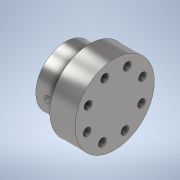
# Autodesk Inventor part: хвостовик
Saved by Autodesk Inventor 2021 (Build 250183000, 183)
## iProperties
Created: 2021-01-19
Part Number: хвостовик
Material: Сталь, легированная
Document SubType Name: ЛистМат
Designer: panda
Density: 7.73 g/cm^3
Sheet Metal Rule: По умолчанию_мм
Appearance: С умеренной полировкой
Mass: 1576.94 g
Surface Area: 253.207 cm^2
Volume: 204.003 cm^3
Author: panda
Autodesk Inventor part; units mm, degrees
ref_plane "YZ Plane" through (0, 0, 0) normal (1, 0, 0) x (0, 1, 0)
ref_plane "XZ Plane" through (0, 0, 0) normal (0, 1, 0) x (-1, 0, 0)
ref_plane "XY Plane" through (0, 0, 0) normal (0, 0, 1) x (1, 0, 0)
sketch "Эскиз1" plane through (0, 0, 0) normal (1, 0, 0) x (0, 1, 0)
  circle A0 centre (0, 0) radius 30.5
  dimension "d0" = 61
  constraints: 1 centre point, 1 coincident
  measures "d0" diameter of A0
extrude "Выдавливание1" add sketch "Эскиз1" along normal blind 25
sketch "Эскиз2" plane through (25, 0, 0) normal (1, 0, 0) x (0, 0, -1)
  circle A0 centre (0, 0) radius 41
  dimension "d3" = 82
  constraints: 1 centre point, 1 coincident
  measures "d3" diameter of A0
extrude "Выдавливание2" add sketch "Эскиз2" along normal blind 26
sketch "Эскиз3" plane through (0, 0, 0) normal (0, 0, 1) x (1, 0, 0)
  line L0 (0, 0) -> (25, 0)
  line L1 (25, -30.5) -> (25, 30.5) projected
  circle A0 centre (12.5, 0) radius 3.5
  dimension "d6" = 7
  constraints: 2 end point, 2 midpoint, 1 centre point
  measures "d6" diameter of A0
extrude "Выдавливание3" cut sketch "Эскиз3" along normal through all both and the other way through all
sketch "Эскиз4" plane through (51, 0, 0) normal (1, 0, 0) x (0, 0, -1)
  circle A0 centre (0, 0) radius 30.5 projected
  line L0 (0, 0) -> (-11.8974, 32.688)
  line L1 (0, 0) -> (0, 6.9467)
  circle A1 centre (-10.4316, 28.6606) radius 4
  line L2 (0, 0) -> (-31.5267, 14.7011)
  circle A2 centre (-27.6424, 12.8899) radius 4
  line L3 (0, 0) -> (-32.688, -11.8974)
  circle A3 centre (-28.6606, -10.4316) radius 4
  line L4 (0, 0) -> (-14.7011, -31.5267)
  circle A4 centre (-12.8899, -27.6424) radius 4
  line L5 (0, 0) -> (11.8974, -32.688)
  circle A5 centre (10.4316, -28.6606) radius 4
  line L6 (0, 0) -> (31.5267, -14.7011)
  circle A6 centre (27.6424, -12.8899) radius 4
  line L7 (0, 0) -> (32.688, 11.8974)
  circle A7 centre (28.6606, 10.4316) radius 4
  line L8 (0, 0) -> (14.7011, 31.5267)
  circle A8 centre (12.8899, 27.6424) radius 4
  dimension "d10" = 20
  dimension "d11" = 8
  dimension "d14" = 360
  constraints: 18 end point, 8 centre point, 8 point on line, 2 coincident, 1 vertical, 41 other
  measures "d10" angle of L0 L1
  measures "d11" diameter of A1
extrude "Выдавливание4" cut sketch "Эскиз4" against normal blind 10 contours A7 L7 A0 | A0 L7 A7 | A6 L6 A0 | A0 L6 A6 | L7 A7 A0 | A0 A7 L7 | L6 A6 A0 | A0 A6 L6 | A8 L8 A0 | A0 L8 A8 | A1 A0 L0 | L0 A0 A1 | A2 A0 L2 | L2 A0 A2 | A3 A0 L3 | L3 A0 A3 | A4 A0 L4 | L4 A0 A4 | A5 A0 L5 | L5 A0 A5 | A8 A0 L8 | A5 L5 A0 | A0 A8 L8 | L0 A1 A0 | A0 A1 L0 | L2 A2 A0 | A0 A2 L2 | L3 A3 A0 | A0 A3 L3 | L4 A4 A0 | A0 A4 L4 | L5 A5 A0
equation "\"Радиус_гибки\" = Толщина"
equation "\"Ширина_просечки\" = Толщина"
equation "\"Глубина_просечки\" = 0.5 * Толщина"
equation "\"Размер_просечки\" = 4 * Толщина"
equation "\"Мин_остаток\" = 2 * Толщина"
equation "\"Радиус_перехода\" = Радиус_гибки"
equation "\"Радиус_Якоби\" = Радиус_гибки"
equation "\"Размер_зазора\" = Толщина"
equation "\"Толщина\" = 0.5"
